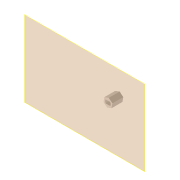
# Autodesk Inventor part: 11_Motor_to_Cassette_Clutch
Saved by Autodesk Inventor 2022 (Build 260153000, 153)
## iProperties
Created: 2023-02-06
Part Number: 11_Motor_to_Cassette_Clutch
Material: Generisch
Document SubType Name: Modeling
Designer: diederichbenedict
Density: 1 g/cm^3
Appearance: Vorgabe
Author: diederichbenedict
Autodesk Inventor part; units mm, degrees
ref_plane "YZ Plane" through (0, 0, 0) normal (1, 0, 0) x (0, 1, 0)
ref_plane "XZ Plane" through (0, 0, 0) normal (0, 1, 0) x (-1, 0, 0)
ref_plane "XY Plane" through (0, 0, 0) normal (0, 0, 1) x (1, 0, 0)
ref_plane "Arbeitsebene1" through (0, 0, 0) normal (0, 0, 1) x (1, 0, 0)
sketch "Skizze1" plane through (0, 0, 0) normal (0, 0, 1) x (1, 0, 0)
  line L0 (66.6303, 35.3317) -> (67.8519, 35.7763) projected
  circle A0 centre (68.575, 31.8892) radius 5.5 projected
  line L1 (65.3022, 34.6354) -> (69.3169, 36.0967)
  line L2 (69.3169, 36.0967) -> (72.5897, 33.3504)
  line L3 (72.5897, 33.3504) -> (71.8478, 29.143)
  line L4 (71.8478, 29.143) -> (67.8331, 27.6817)
  line L5 (67.8331, 27.6817) -> (64.5603, 30.428)
  line L6 (64.5603, 30.428) -> (65.3022, 34.6354)
  arc A1 (66.575, 33.3892) -> (66.075, 31.8892) centre (68.575, 31.8892) ccw projected
  line L7 (70.575, 33.3892) -> (66.575, 33.3892) projected
  arc A2 (71.075, 31.8892) -> (70.575, 33.3892) centre (68.575, 31.8892) ccw projected
  arc A3 (70.575, 30.3892) -> (71.075, 31.8892) centre (68.575, 31.8892) ccw projected
  line L8 (66.575, 30.3892) -> (70.575, 30.3892) projected
  arc A4 (66.075, 31.8892) -> (66.575, 30.3892) centre (68.575, 31.8892) ccw projected
  arc A5 (66.5256, 33.4892) -> (65.975, 31.8892) centre (68.575, 31.8892) ccw
  arc A6 (65.975, 31.8892) -> (66.5256, 30.2892) centre (68.575, 31.8892) ccw
  line L9 (66.5256, 30.2892) -> (70.6244, 30.2892)
  arc A7 (70.6244, 30.2892) -> (71.175, 31.8892) centre (68.575, 31.8892) ccw
  arc A8 (71.175, 31.8892) -> (70.6244, 33.4892) centre (68.575, 31.8892) ccw
  line L10 (70.6244, 33.4892) -> (66.5256, 33.4892)
  point P0 (0, 0)
  dimension "d0" = 0.2
  dimension "d3" = 0.1
  constraints: 16 end point, 8 point on circle, 4 centre point, 1 coincident, 1 parallel, 18 other
  measures "d0" distance between parallel lines of L1 L0
  measures "d3" distance between parallel lines of L7 L10
extrude "Extrusion1" add sketch "Skizze1" against normal blind 10 contours L1 L2 L3 L4 L5 L6
